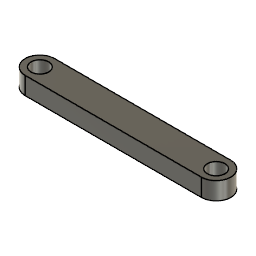
Engine assembly (Autodesk Fusion 360 archive; units mm, degrees)
design "Connecting rod"
part number: 2026-07-12-13-30-28-527
Autodesk Fusion 360 part; units mm, degrees
sketch "Sketch6" plane through (0, 0, 0) normal (0, 0, 1) x (1, 0, 0)
  line L0 (0, -5) -> (60, -5)
  arc A0 (60, -5) -> (60, 5) centre (60, 0) ccw
  line L1 (60, 5) -> (0, 5)
  arc A1 (0, 5) -> (0, -5) centre (0, 0) ccw
  line L2 (0, 0) -> (60, 0) construction
  dimension "d13" = 10
  dimension "d14" = 60
  constraint tangent L0 A0
  constraint tangent A0 L1
  constraint parallel L0 L1
  constraint tangent L1 A1
  constraint tangent L0 A1
  constraint horizontal L2
  constraint coincident A1.centre L2.start
  measures "d13" diameter of A0
  measures "d14" distance of A1.centre A0.centre
extrude "Extrude4" add sketch "Sketch6" along normal blind 6
sketch "Sketch7" plane through (0, 0, 6) normal (0, 0, 1) x (-1, 0, 0)
  arc A0 (0, -5) -> (0, 5) centre (0, 0) ccw
  line L0 (0, 5) -> (-60, 5)
  arc A1 (-60, 5) -> (-60, -5) centre (-60, 0) ccw
  line L1 (-60, -5) -> (0, -5)
  circle A2 centre (0, 0) radius 3
  circle A3 centre (-60, 0) radius 3
  dimension "d17" = 6
  dimension "d18" = 6
  constraint coincident A0.centre A2.centre
  constraint concentric A1 A3
  measures "d17" diameter of A2
  measures "d18" diameter of A3
extrude "Extrude5" cut sketch "Sketch7" against normal blind 10 contours A2 | A3

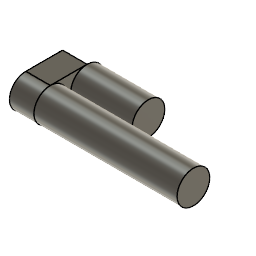
design "Crankshaft"
part number: 2026-07-12-13-02-29-244
Autodesk Fusion 360 part; units mm, degrees
sketch "Sketch1" plane through (0, 0, 0) normal (1, 0, 0) x (0, 1, 0)
  circle A0 centre (0, 0) radius 4
  dimension "d1" = 8
  constraint coincident A0.centre origin
  measures "d1" diameter of A0
extrude "Extrude1" add sketch "Sketch1" along normal blind 15 makes body 1
sketch "Sketch2" plane through (0, 0, 0) normal (1, 0, 0) x (0, 1, 0)
  circle A0 centre (-9, 0) radius 4
  dimension "d4" = 8
  measures "d4" diameter of A0
extrude "Extrude2" add sketch "Sketch2" along normal blind 20 separate body makes body 2
sketch "Sketch3" plane through (0, 0, 0) normal (-1, 0, 0) x (0, -1, 0)
  circle A0 centre (0, 0) radius 4
  line L0 (0, -4) -> (9, -4)
  arc A1 (9, -4) -> (9, 4) centre (9, 0) ccw
  line L1 (9, 4) -> (0, 4)
  arc A2 (0, 4) -> (0, -4) centre (0, 0) ccw
  line L2 (0, 0) -> (9, 0) construction
  dimension "d7" = 8
  constraint tangent L0 A1
  constraint tangent A1 L1
  constraint parallel L0 L1
  constraint tangent L1 A2
  constraint tangent L0 A2
  constraint horizontal L2
  constraint coincident A0.centre A2.centre
  measures "d7" diameter of A1
extrude "Extrude3" add sketch "Sketch3" along normal blind 6 separate body contours A0 L0 A1 L1 makes body 3
sketch "Sketch4" plane through (20, 0, 0) normal (1, 0, 0) x (0, 1, 0)
  circle A0 centre (-9, 0) radius 4
  circle A1 centre (-9, 0) radius 4
  dimension "d10" = 8
  constraint concentric A0 A1
  measures "d10" diameter of A1
extrude "Extrude4" add sketch "Sketch4" along normal blind 15 bodies 2

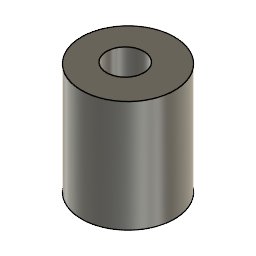
design "Piston"
part number: 2026-07-12-14-23-25-142
Autodesk Fusion 360 part; units mm, degrees
sketch "Sketch1" plane through (0, 0, 0) normal (0, 0, 1) x (1, 0, 0)
  circle A0 centre (0, 0) radius 12.5
  dimension "d1" = 25
  constraint coincident A0.centre origin
  measures "d1" diameter of A0
extrude "Extrude1" add sketch "Sketch1" along normal blind 30
ref_plane "WorkPlane1" through (0, 0, 15) normal (0, 0, 1) x (1, 0, 0)
sketch "Sketch2" plane through (0, 0, 15) normal (0, 0, 1) x (1, 0, 0)
  circle A0 centre (-0.7442, 0) radius 5
  dimension "d6" = 10
  measures "d6" diameter of A0
extrude "Extrude2" cut sketch "Sketch2" along normal blind 20 and the other way blind 20
